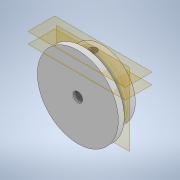
# Autodesk Inventor part: Encoder_Mount3_Wheel
Saved by Autodesk Inventor 2022 (Build 260153000, 153)
## iProperties
Created: 2024-04-30
Part Number: Encoder_Mount3_Wheel
Material: Generic
Document SubType Name: Modeling
Designer: Gotham City
Density: 1 g/cm^3
Appearance: Default
Author: Gotham City
Autodesk Inventor part; units mm, degrees
ref_plane "YZ Plane" through (0, 0, 0) normal (1, 0, 0) x (0, 1, 0)
ref_plane "XY Plane" through (0, 0, 0) normal (0, 0, 1) x (1, 0, 0)
sketch "Sketch1" plane through (0, 0, 0) normal (0, 0, 1) x (1, 0, 0)
  circle A0 centre (0, 0) radius 9
  dimension "d0" = 18
  constraints: 1 centre point, 1 coincident
  measures "d0" diameter of A0
extrude "Extrusion1" add sketch "Sketch1" along normal blind 5
sketch "Sketch2" plane through (0, 0, 5) normal (0, 0, 1) x (1, 0, 0)
  circle A0 centre (0, 0) radius 11
  circle A1 centre (0, 0) radius 9 projected
  dimension "d3" = 2
  constraints: 1 centre point, 1 coincident
  measures "d3" radial gap between concentric circles of A0 A1
extrude "Extrusion2" add sketch "Sketch2" along normal blind 1.6 contours A0 | A1
ref_plane "Work Plane1" through (0, 0, 2.5) normal (0, 0, 1) x (1, 0, 0)
sketch "Sketch3" plane through (0, 0, 2.5) normal (0, 0, 1) x (1, 0, 0)
  circle A0 centre (0, 0) radius 9 projected
  point P0 (0, 9)
  constraints: 1 vertical alignment, 1 other
ref_plane "Work Plane2" through (0, 9, 2.5) normal (0, 1, 0) x (-1, 0, 0)
sketch "Sketch4" plane through (0, 9, 2.5) normal (0, 1, 0) x (-1, 0, 0)
  point P0 (0, -2.5)
  point P1 (0, 0)
hole "Hole1" at (0, 9, 2.5) direction (0, -1, 0) diameter 2.1 depth 6 tip angle 118 clearance for "Socket Head Cap Screw ISO 4762" size "M2" standard "ISO"
ref_plane "Work Plane3" through (0, 6, 2.5) normal (0, 1, 0) x (-1, 0, 0)
sketch "Sketch5" plane through (0, 6, 2.5) normal (0, 1, 0) x (-1, 0, 0)
  circle A0 centre (0, 0) radius 1.05 projected
  line L0 (2.05, 1.1836) -> (2.05, -1.1836)
  line L1 (2.05, -1.1836) -> (0, -2.3671) construction
  line L2 (0, -2.3671) -> (-2.05, -1.1836) construction
  line L3 (-2.05, -1.1836) -> (-2.05, 1.1836)
  line L4 (-2.05, 1.1836) -> (0, 2.3671)
  line L5 (0, 2.3671) -> (2.05, 1.1836)
  line L6 (2.05, -1.1836) -> (2.05, -2.5)
  line L7 (9, -2.5) -> (-9, -2.5) projected
  line L8 (-2.05, -1.1836) -> (-2.05, -2.5)
  point P0 (0, -2.5)
  dimension "d14" = 4.1
  constraints: 16 end point, 2 point on line, 2 vertical, 1 coincident, 1 perpendicular, 13 other
  measures "d14" distance between parallel lines of L3 L0
extrude "Extrusion3" cut sketch "Sketch5" against normal blind 1.65
sketch "Sketch6" plane through (0, 0, 6.6) normal (0, 0, 1) x (1, 0, 0)
  circle A0 centre (0, 0) radius 3.0931 construction
  constraints: 2 coincident, 1 centre point
hole "Hole3" at (0, 0, 6.6) direction (0, 0, -1) diameter 2.6 end through all clearance for "Socket Head Cap Screw ISO 4762" size "M2.5" standard "ISO"
body "Solid1"
